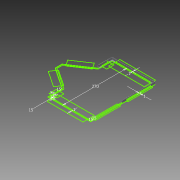
# Autodesk Inventor part: male
Saved by Autodesk Inventor 2015 (Build 190159000, 159)
## iProperties
Created: 2016-08-08
Part Number: male
Material: Generic
Document SubType Name: Modeling
Designer: Javier
Density: 1 g/cm^3
Appearance: Default
Author: Javier
Autodesk Inventor part; units mm, degrees
ref_plane "YZ Plane" through (0, 0, 0) normal (1, 0, 0) x (0, 1, 0)
ref_plane "XZ Plane" through (0, 0, 0) normal (0, 1, 0) x (-1, 0, 0)
ref_plane "XY Plane" through (0, 0, 0) normal (0, 0, 1) x (1, 0, 0)
sketch "Sketch1" plane through (0, 0, 0) normal (0, 1, 0) x (-1, 0, 0)
  line L0 (82.171, 116.0061) -> (-97.829, 116.0061)
  line L1 (-97.829, 116.0061) -> (-97.829, -153.9939)
  line L2 (-97.829, -153.9939) -> (82.171, -153.9939)
  line L3 (81.171, 115.0061) -> (-96.829, 115.0061)
  line L4 (-96.829, 115.0061) -> (-96.829, -152.9939)
  line L5 (-96.829, -152.9939) -> (81.171, -152.9939)
  line L6 (81.171, 56.2728) -> (81.171, 115.0061)
  line L7 (82.171, -153.9939) -> (82.171, -93.7272)
  line L8 (82.171, 55.7393) -> (82.171, 116.0061)
  line L9 (81.171, -152.9939) -> (81.171, -94.2607)
  line L10 (-92.829, 111.0061) -> (77.171, 111.0061)
  line L11 (-92.829, 111.0061) -> (-92.829, -148.9939)
  line L12 (-92.829, -148.9939) -> (77.171, -148.9939)
  line L13 (77.171, 111.0061) -> (77.171, 58.4069)
  line L14 (77.171, -96.3948) -> (77.171, -148.9939)
  line L15 (67.171, 133.2815) -> (-82.829, 133.2815)
  line L16 (-82.829, 133.2815) -> (-82.829, 85.6394)
  line L17 (-82.829, 85.6394) -> (67.171, 85.6394)
  line L18 (67.171, 85.6394) -> (67.171, 133.2815)
  line L19 (91.8793, 101.0061) -> (59.7353, 101.0061)
  line L20 (59.7353, 101.0061) -> (59.7353, 70.7393)
  line L21 (59.7353, 70.7393) -> (91.8793, 70.7393)
  line L22 (91.8793, 70.7393) -> (91.8793, 101.0061)
  line L23 (-88.3298, 101.0061) -> (-103.1355, 101.0061)
  line L24 (-103.1355, 101.0061) -> (-103.1355, -3.9939)
  line L25 (-103.1355, -3.9939) -> (-88.3298, -3.9939)
  line L26 (-88.3298, -3.9939) -> (-88.3298, 101.0061)
  line L27 (67.171, -171.2694) -> (-82.829, -171.2694)
  line L28 (-82.829, -171.2694) -> (-82.829, -123.6273)
  line L29 (-82.829, -123.6273) -> (67.171, -123.6273)
  line L30 (67.171, -123.6273) -> (67.171, -171.2694)
  line L31 (91.8793, -138.9939) -> (59.7353, -138.9939)
  line L32 (59.7353, -138.9939) -> (59.7353, -108.7272)
  line L33 (59.7353, -108.7272) -> (91.8793, -108.7272)
  line L34 (91.8793, -108.7272) -> (91.8793, -138.9939)
  line L35 (-88.3298, -138.9939) -> (-103.1355, -138.9939)
  line L36 (-103.1355, -138.9939) -> (-103.1355, -33.9939)
  line L37 (-103.1355, -33.9939) -> (-88.3298, -33.9939)
  line L38 (-88.3298, -33.9939) -> (-88.3298, -138.9939)
  line L39 (82.171, 55.7393) -> (171.671, -4.2607)
  line L40 (82.171, -93.7272) -> (171.671, -33.7272)
  line L41 (171.671, -4.2607) -> (171.671, -33.7272)
  line L42 (90.3045, 40.9341) -> (157.1017, -3.8462)
  line L43 (107.5303, 66.6293) -> (174.3275, 21.8491)
  line L44 (107.5303, 66.6293) -> (90.3045, 40.9341)
  line L45 (174.3275, 21.8491) -> (157.1017, -3.8462)
  line L46 (174.3275, -59.837) -> (157.1017, -34.1417)
  line L47 (107.5303, -104.6172) -> (174.3275, -59.837)
  line L48 (90.3045, -78.922) -> (157.1017, -34.1417)
  line L49 (107.5303, -104.6172) -> (90.3045, -78.922)
  line L50 (170.671, -4.7942) -> (170.671, -33.1937)
  line L51 (166.671, -6.9284) -> (166.671, -31.0595)
  line L52 (166.671, -6.9284) -> (77.171, 53.0716)
  line L53 (81.171, 56.2728) -> (81.171, 55.2058)
  line L54 (77.171, 58.4069) -> (77.171, 53.0716)
  line L55 (170.671, -4.7942) -> (81.171, 55.2058)
  line L56 (35.7741, 85.6394) -> (35.6306, 85.7356)
  line L57 (166.671, -31.0595) -> (77.171, -91.0595)
  line L58 (81.171, -94.2607) -> (81.171, -93.1937)
  line L59 (77.171, -96.3948) -> (77.171, -91.0595)
  line L60 (170.671, -33.1937) -> (81.171, -93.1937)
  dimension "d0" = 270
  dimension "d3" = 1
  dimension "d4" = 1
  dimension "d5" = 1
  dimension "d17" = 5
  dimension "d30" = 5
  dimension "d31" = 1
  dimension "d32" = 15
  dimension "d33" = 15
  dimension "d34" = 15
  dimension "d35" = 15
  dimension "d38" = 15
  constraints: 122 end point, 16 parallel, 7 horizontal, 6 vertical, 5 perpendicular, 1 point on line
  measures "d0" distance between parallel lines of L2 L0
  measures "d3" distance between parallel lines of L2 L5
  measures "d4" distance between parallel lines of L1 L4
  measures "d5" distance between parallel lines of L3 L0
  measures "d17" distance between parallel lines of L0 L10
  measures "d30" distance between parallel lines of L13 L8
  measures "d31" distance between parallel lines of L6 L8
  measures "d32" distance from line of L21 L8.start
  measures "d33" distance between parallel lines of L0 L19
  measures "d34" distance between parallel lines of L18 L8
  measures "d35" distance between parallel lines of L1 L16
  measures "d38" distance between parallel lines of L23 L0
extrude "Extrusion1" add sketch "Sketch1" along normal blind 10 contours L8 L19 L6 L3 L18 L0 | L18 L3 L16 L0 | L8 L21 L6 L19 | L16 L3 L4 L23 L1 L0 | L8 L39 L44 L55 L53 L6 L21 | L23 L4 L25 L1 | L39 L45 L55 L44 | L25 L4 L37 L1 | L39 L41 L40 L46 L60 L50 L55 L45 | L37 L4 L35 L1 | L35 L4 L5 L28 L2 L1 | L40 L49 L60 L46 | L28 L5 L30 L2 | L40 L7 L33 L9 L58 L60 L49 | L30 L5 L9 L31 L7 L2 | L7 L31 L9 L33
extrude "Extrusion2" add sketch "Sketch1" along normal blind 1 contours L18 L10 L16 L3 | L3 L6 L19 L13 L10 L18 | L6 L21 L13 L19 | L16 L10 L11 L23 L4 L3 | L6 L53 L55 L44 L52 L54 L13 L21 | L23 L11 L25 L4 | L55 L45 L52 L44 | L25 L11 L37 L4 | L55 L50 L60 L46 L57 L51 L52 L45 | L37 L11 L35 L4 | L35 L11 L12 L28 L5 L4 | L60 L49 L57 L46 | L28 L12 L30 L5 | L60 L58 L9 L33 L14 L59 L57 L49 | L30 L12 L14 L31 L9 L5 | L9 L31 L14 L33
fillet "Fillet1" radius 1 8 edges at (-81.171, 1, -123.0938) (7.829, 1, -152.9939) (-81.171, 1, 85.1059) (7.829, 1, 115.0061) (96.829, 1, -18.9939) (-125.921, 1, -63.1937) (-170.671, 1, -18.9939) (-125.921, 1, 25.2058)
extrude "Extrusion5" cut sketch "Sketch1" along normal blind 7.5 contours L18 L3 L16 L0 | L0 L16 L15 L18 | L19 L22 L21 L8 | L8 L21 L6 L19 | L18 L10 L16 L3 | L6 L21 L13 L19 | L18 L19 L20 L17 L16 L10 | L13 L21 L20 L17 L18 L19 | L23 L4 L25 L1 | L1 L25 L24 L23 | L18 L17 L20 L19 | L44 L43 L45 L39 | L39 L45 L55 L44 | L23 L11 L25 L4 | L55 L45 L52 L44 | L37 L4 L35 L1 | L1 L35 L36 L37 | L23 L26 L25 L11 | L52 L45 L42 L44 | L37 L11 L35 L4 | L37 L38 L35 L11 | L46 L47 L49 L40 | L40 L49 L60 L46 | L28 L5 L30 L2 | L2 L30 L27 L28 | L60 L49 L57 L46 | L28 L12 L30 L5 | L57 L49 L48 L46 | L28 L29 L32 L31 L30 L12 | L33 L34 L31 L7 | L7 L31 L9 L33 | L9 L31 L14 L33 | L31 L32 L29 L30 | L30 L29 L32 L33 L14 L31
sketch "Sketch3" plane through (0, 10, 0) normal (0, 1, 0) x (1, 0, 0)
  line L0 (-77.171, -53.0716) -> (-77.171, 91.0595)
  line L1 (-77.171, 91.0595) -> (-82.171, 93.7272)
  line L2 (-82.171, 93.7272) -> (-237.6798, 93.7272)
  line L3 (-237.6798, 93.7272) -> (-237.6798, -55.7393)
  line L4 (-80.171, -70.7393) -> (-80.171, -54.6722) projected
  line L5 (-77.171, -53.0716) -> (-82.171, -55.7393)
  line L6 (-82.171, -55.7393) -> (-237.6798, -55.7393)
  line L7 (-77.171, 18.9939) -> (139.9462, 18.9939)
  line L8 (139.9462, 18.9939) -> (139.9462, 278.7318)
  line L9 (139.9462, 278.7318) -> (-77.171, 278.7318)
  line L10 (-126.7833, 93.7272) -> (-77.171, 278.7318)
  point P0 (0, 0)
  point P1 (-81.171, -55.2058)
  constraints: 20 end point, 3 perpendicular, 2 horizontal, 1 midpoint, 1 parallel, 1 point on line, 1 vertical
extrude "Extrusion9" cut sketch "Sketch3" against normal blind 100 contours L0 L1 L2 L10 L9 L8 L7 keep common part
sketch "Sketch6" plane through (96.829, 10, -18.9939) normal (0, 0, 1) x (1, 0, 0)
  line L0 (1, -10) -> (-4, -10)
  line L1 (-4, -10) -> (-4, -2.5)
  line L2 (-4, -2.5) -> (1, -2.5)
  line L3 (1, -2.5) -> (1, -10)
  point P0 (-96.829, -10)
  dimension "d68" = 7.5
  dimension "d69" = 5
  constraints: 8 end point, 2 parallel, 1 horizontal, 1 perpendicular
  measures "d68" distance between parallel lines of L0 L2
  measures "d69" distance between parallel lines of L3 L1
extrude "Extrusion10" add sketch "Sketch6" against normal blind 1
sketch "Sketch7" plane through (-82.171, 0, -93.7272) normal (-0.4707228, 0, 0.8822811) x (0.8822811, 0, 0.4707228)
  line L0 (117.2074, 7.5) -> (-15.1347, 7.5) projected
  line L1 (0, 0) -> (5.6671, 0)
  line L2 (5.6671, 0) -> (5.6671, 7.5)
  line L3 (5.6671, 7.5) -> (0, 7.5)
  line L4 (0, 7.5) -> (0, 0)
  point P0 (116.6174, 0)
  constraints: 8 end point, 2 parallel, 1 horizontal, 1 perpendicular, 1 point on line
extrude "Extrusion11" add sketch "Sketch7" against normal blind 1
body "Solid1"
